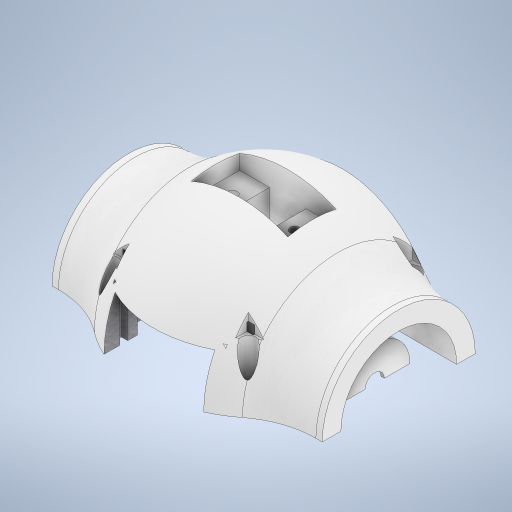
# Autodesk Inventor part: body front moter middle lemon shape for printing
Saved by Autodesk Inventor 2023 (Build 270158000, 158)
## iProperties
Created: 2022-10-08
Part Number: body front moter middle lemon shape for printing
Material: ABS プラスチック
Document SubType Name: Modeling
Designer: ellie
Density: 1.06 g/cm^3
Appearance: 積雪
Author: ellie
Autodesk Inventor part; units mm, degrees
ref_plane "YZ Plane" through (0, 0, 0) normal (1, 0, 0) x (0, 1, 0)
ref_plane "XZ Plane" through (0, 0, 0) normal (0, 1, 0) x (-1, 0, 0)
ref_plane "XY Plane" through (0, 0, 0) normal (0, 0, 1) x (1, 0, 0)
sketch "スケッチ1" plane through (0, 0, 0) normal (0, 1, 0) x (-1, 0, 0)
  circle A0 centre (0, 0) radius 37.5
  line L0 (0, 0) -> (0, -37.5)
  line L1 (0, 0) -> (0, 37.5)
  dimension "d0" = 75
  constraints: 4 end point, 2 point on circle, 2 vertical, 1 centre point, 1 coincident
  measures "d0" diameter of A0
revolve "回転1" add sketch "スケッチ1" angle 180 about axis through (0, 0, 0) along (0, 0, 1) picked at (-2.7815, -24.6866) contours L1 L0 A0
sketch "スケッチ5" plane through (0, 0, 0) normal (0, -1, 0) x (1, 0, 0)
  line L0 (-21, -21) -> (21, -21)
  line L1 (21, -21) -> (21, -9)
  line L2 (21, -9) -> (-21, -9)
  line L3 (-21, -9) -> (-21, -21)
  line L4 (-21, -11) -> (-21, -9)
  line L5 (0, 29.25) -> (-17.5, 29.25)
  line L6 (-17.5, 29.25) -> (-17.5, 26.75)
  line L7 (-17.5, 26.75) -> (0, 26.75)
  line L8 (0, 26.75) -> (0, 29.25)
  line L9 (0, 23.75) -> (-20.5, 23.75)
  line L10 (-20.5, 23.75) -> (-20.5, 22.25)
  line L11 (-20.5, 22.25) -> (0, 22.25)
  line L12 (0, 22.25) -> (0, 23.75)
  line L13 (0, 16.25) -> (-21.5, 16.25)
  line L14 (-21.5, 16.25) -> (-21.5, 13.75)
  line L15 (-21.5, 13.75) -> (0, 13.75)
  line L16 (0, 13.75) -> (0, 16.25)
  line L17 (0, 7.75) -> (-24, 7.75)
  line L18 (-24, 7.75) -> (-24, 5.25)
  line L19 (-24, 5.25) -> (0, 5.25)
  line L20 (0, 5.25) -> (0, 7.75)
  circle A0 centre (0, 0) radius 37.5 projected
  circle A1 centre (0, 0) radius 37.5 projected
  line L21 (0, 37.5) -> (0, -37.5)
  line L22 (37.5, 0) -> (-37.5, 0)
  line L23 (-33.5, 5.25) -> (-24, 5.25)
  line L24 (-24, 5.25) -> (-24, -5.25)
  line L25 (-24, -5.25) -> (-33.5, -5.25)
  line L26 (-33.5, -5.25) -> (-33.5, 5.25)
  line L27 (-24, -8.0262) -> (-24, 5.25)
  line L28 (-29, 23.775) -> (-29, -23.775)
  line L29 (-15.5, 29.25) -> (0, 29.25)
  line L30 (0, 29.25) -> (0, 37.5)
  line L31 (0, 37.5) -> (-15.5, 37.5)
  line L32 (-15.5, 37.5) -> (-15.5, 29.25)
  line L33 (-15.5, 26.75) -> (0, 26.75)
  line L34 (0, 26.75) -> (0, 23.75)
  line L35 (0, 23.75) -> (-15.5, 23.75)
  line L36 (-15.5, 23.75) -> (-15.5, 26.75)
  line L37 (-19, 16.25) -> (0, 16.25)
  line L38 (0, 16.25) -> (0, 22.25)
  line L39 (0, 22.25) -> (-19, 22.25)
  line L40 (-19, 22.25) -> (-19, 16.25)
  line L41 (-19, 13.75) -> (0, 13.75)
  line L42 (0, 13.75) -> (0, 7.75)
  line L43 (0, 7.75) -> (-19, 7.75)
  line L44 (-19, 7.75) -> (-19, 13.75)
  line L45 (-24, 0) -> (-40.9365, 0)
  line L46 (-24, 0) -> (-9.0837, 0)
  line L47 (-9, 5.25) -> (-24, 5.25)
  line L48 (-24, 5.25) -> (-24, -5.25)
  line L49 (-24, -5.25) -> (-9, -5.25)
  line L50 (-9, 5.25) -> (-24, -5.25) construction
  line L51 (-24, 5.25) -> (-9, -5.25) construction
  line L52 (-24, 7.25) -> (-34.5, 7.25)
  line L53 (-34.5, 7.25) -> (-34.5, -7.25)
  line L54 (-34.5, -7.25) -> (-24, -7.25)
  line L55 (-24, -7.25) -> (-24, 7.25)
  line L56 (-24, 7.25) -> (-34.5, -7.25) construction
  line L57 (-34.5, 7.25) -> (-24, -7.25) construction
  line L58 (-8.35, 5.25) -> (-1, 5.25)
  line L59 (-1, 5.25) -> (-1, -5.25)
  line L60 (-1, -5.25) -> (-8.35, -5.25)
  line L61 (-8.35, 5.25) -> (-1, -5.25) construction
  line L62 (-1, 5.25) -> (-8.35, -5.25) construction
  line L63 (-24, 5.25) -> (-29, 5.25)
  line L64 (-24, -5.25) -> (-29, -5.25)
  line L65 (-24, 7.25) -> (-29, 7.25)
  line L66 (-24, -7.25) -> (-29, -7.25)
  line L67 (28.3901, -24.5) -> (-28.3901, -24.5)
  line L68 (-8.35, 5.25) -> (-6.8, 5.25)
  line L69 (-6.6281, -5.25) -> (-7.8281, -5.25)
  line L70 (0, 7.75) -> (1, 7.75)
  line L71 (0, -3) -> (0, 7.75)
  line L72 (-12.5791, -9) -> (-9, -9)
  line L73 (-1, -5.25) -> (-24, -5.25)
  point P0 (0, -21)
  point P1 (0, -9)
  point P2 (0, 28)
  point P3 (0, 23)
  point P4 (0, 15)
  point P5 (0, 6.5)
  point P6 (-21, -15)
  point P7 (-27, -0.5262)
  point P8 (-29, -5.25)
  point P9 (-15.5, 25.25)
  point P10 (-15.5, 34.1467)
  point P11 (0, 29.25)
  point P12 (0, 26.75)
  point P13 (0, 13.75)
  point P14 (0, 16.25)
  point P15 (-29, 0)
  point P16 (-33.5, 0)
  point P17 (-24, 0)
  point P18 (-16.5, 0)
  point P19 (-29.25, 0)
  point P20 (-4.675, 0)
  point P21 (-27, 0.5)
  point P22 (-28, 0.4738)
  point P23 (-28, -11.5262)
  point P24 (-27, -11.5)
  point P25 (-24, -5.25)
  point P26 (-24, -5.25)
  point P27 (-24, -5.25)
  point P28 (-24, 5.25)
  point P29 (-24, -5.25)
  point P30 (-1, 0)
  point P31 (-8, 5.25)
  point P32 (-8, -5.25)
  point P33 (0, 5.25)
  point P34 (-29, -7.25)
  point P35 (-29, 7.25)
  point P36 (-24, -1.3881)
  point P37 (-9, -5.25)
  dimension "d12" = 42
  dimension "d13" = 12
  dimension "d23" = 17.5
  dimension "d24" = 2.5
  dimension "d27" = 20.5
  dimension "d28" = 1.5
  dimension "d30" = 21.5
  dimension "d31" = 2.5
  dimension "d33" = 2.5
  dimension "d88" = 0
  dimension "d89" = 0
  dimension "d90" = 16.5
  dimension "d92" = 21
  dimension "d97" = 9.5
  dimension "d98" = 10.5
  dimension "d113" = 29
  dimension "d122" = 15.5
  dimension "d124" = 3
  dimension "d125" = 15.5
  dimension "d126" = 6
  dimension "d127" = 6
  dimension "d161" = 14.5
  dimension "d162" = 10.5
  dimension "d164" = 10.5
  dimension "d170" = 24.5
  dimension "d187" = 1
  dimension "d283" = 23
  dimension "d284" = 10.5
  dimension "d285" = 15
  dimension "d286" = 34.5
  dimension "d287" = 1
  dimension "d288" = 19
  dimension "d289" = 19
  constraints: 146 end point, 26 parallel, 19 horizontal, 16 midpoint, 16 perpendicular, 15 point on line, 9 collinear, 1 vertical, 20 other
  measures "d12" distance of L2.end L1.end
  measures "d13" distance of L1.end L0.end
  measures "d23" distance of L7.end L6.end
  measures "d24" distance of L6.end L5.end
  measures "d27" distance of L11.end L10.end
  measures "d28" distance of L10.end L9.end
  measures "d30" distance of L15.end L14.end
  measures "d31" distance of L14.end L13.end
  measures "d33" distance of L18.end L17.end
  measures "d89" distance from line of point (0, 0) L22
  measures "d90" distance from line of L0 point (0, -37.5)
  measures "d92" distance of the line from the sketch origin of L3
  measures "d97" distance of L24.end L25.end
  measures "d98" distance of L23.end L24.end
  measures "d113" distance of the line from the sketch origin of L28
  measures "d122" distance of the line from the sketch origin of L32
  measures "d124" distance of L33.end L34.end
  measures "d126" distance of L38.end L37.end
  measures "d127" distance of L41.end L42.end
  measures "d161" distance between parallel lines of L54 L52
  measures "d162" distance between parallel lines of L48 L53
  measures "d164" distance between parallel lines of L60 L58
  measures "d170" distance between parallel lines of L67 L22
  measures "d187" distance between parallel lines of L71 L59
  measures "d283" distance between parallel lines of L55 L59
  measures "d284" distance between parallel lines of L49 L47
  measures "d285" distance of L48.end L49.end
  measures "d286" distance of the line from the sketch origin of L53
  measures "d287" distance of the line from the sketch origin of L59
  measures "d288" distance of the line from the sketch origin of L40
  measures "d289" distance of the line from the sketch origin of L44
extrude "GNSボード" cut sketch "スケッチ5" against normal blind 16.5 contours L8 L7 L6 L5
extrude "GNSボード止めるよう" cut sketch "スケッチ5" against normal blind 15 contours L21 L5 L32 A0 | L21 L9 L36 L7
extrude "アルミ板１" cut sketch "スケッチ5" against normal blind 20.5 contours L12 L11 L10 L9
extrude "メイン基板" cut sketch "スケッチ5" against normal blind 21.5 contours L15 L14 L13 L16
extrude "メイン止めるよう" cut sketch "スケッチ5" against normal blind 16.5 contours L17 L44 L15 L21 | L13 L40 L11 L21
extrude "アルミ板２" cut sketch "スケッチ5" against normal blind 20.5 contours L19 L18 L17 L20
extrude "電池ボックス入れ" cut sketch "スケッチ5" against normal blind 13 contours L3 L2 L21 L0 | L21 L2 L1 L0
extrude "side ut" cut sketch "スケッチ5" against normal blind 100 contours A0 L22 L53 L54 L28 | A0 L28 L52 L53 L22 | L54 L53 L22 L26 L25 L28 | L53 L52 L28 L23 L26 L22 | L25 L26 L22 L28 | L26 L23 L28 L22
extrude "motor case" add sketch "スケッチ5" against normal blind 7 contours L54 L53 L22 L26 L25 L28 | L28 L25 L27 L54 | L53 L52 L28 L23 L26 L22 | L28 L22 L24 L25 | L25 L26 L22 L28 | L22 L28 L23 L24 | L52 L18 L23 L28 | L26 L23 L28 L22
extrude "bottom cut" cut sketch "スケッチ5" against normal blind 90 contours L67 A0 L21 | L21 A0 L67
extrude "motor" cut sketch "スケッチ5" against normal blind 6 contours L28 L22 L24 L25 | L25 L26 L22 L28 | L22 L28 L23 L24 | L26 L23 L28 L22
extrude "motor block" cut sketch "スケッチ5" against normal up to surface (6 mm away) contours L59 L60 L73 L49 L24 L22 | L22 L24 L19 L59
sketch "スケッチ26" plane through (-34.5, 0, -7.25) normal (-1, 0, 0) x (0, 0, 1)
  line L0 (14.5, 0) -> (0, 0) projected
  circle A0 centre (7.25, 0) radius 3
  point P0 (7.25, 0)
  point P1 (7.25, 0)
  point P2 (4.25, 0)
  point P3 (10.25, 0)
  dimension "d197" = 6
  constraints: 1 centre point, 1 coincident
  measures "d197" diameter of A0
extrude "押し出し34" cut sketch "スケッチ26" against normal blind 27 contours L0 A0 picked at (7.9985, 0.6631)
mirror "ミラー11" about plane through (0, 0, 0) normal (1, 0, 0) of "GNSボード", "GNSボード止めるよう", "アルミ板１", "メイン止めるよう", "メイン基板", "アルミ板２", "motor", "押し出し34", "motor case", "電池ボックス入れ", "motor block", "side ut"
ref_plane "作業平面5" through (0, 13, 0) normal (0, -1, 0) x (1, 0, 0)
ref_plane "作業平面6" through (-15.5, 37, 29.25) normal (0, -1, 0) x (1, 0, 0)
sketch "スケッチ29" plane through (-15.5, 37, 29.25) normal (0, -1, 0) x (1, 0, 0)
  line L0 (15.5, -29.25) -> (-67.7134, -29.25)
  line L1 (-67.7134, -29.25) -> (15.5, -29.25)
  line L2 (110.7852, -24.5555) -> (110.7852, -27.3413)
  line L3 (15.5, -29.25) -> (98.1975, -29.25)
  circle A0 centre (25.2, -29.25) radius 1.5
  circle A1 centre (5.8, -29.25) radius 1.5
  line L4 (32.1864, 0) -> (-1.1864, 0) projected
  line L5 (15.5, 0) -> (15.5, -53.75)
  line L6 (-12.8901, -53.75) -> (43.8901, -53.75) projected
  point P0 (32.5, 0)
  point P1 (-1.5, 0)
  point P2 (43.8901, -53.75)
  point P3 (-11.5, -52)
  point P4 (42.5, -52)
  dimension "d205" = 3
  dimension "d206" = 19.4
  dimension "d207" = 0
  constraints: 10 end point, 2 centre point, 2 horizontal, 1 collinear, 1 midpoint, 1 vertical, 3 other
  measures "d205" diameter of A0
  measures "d206" distance of A1.centre A0.centre
  measures "d207" distance from line of L3 A0.centre
extrude "押し出し36" cut sketch "スケッチ29" along normal blind 25
sketch "スケッチ30" plane through (-15.5, 37, 29.25) normal (0, -1, 0) x (1, 0, 0)
  line L0 (0.5, -21.75) -> (30.5, -21.75)
  line L1 (30.5, -21.75) -> (30.5, -36.75)
  line L2 (30.5, -36.75) -> (0.5, -36.75)
  line L3 (0.5, -36.75) -> (0.5, -21.75)
  line L4 (0.5, -21.75) -> (30.5, -36.75) construction
  line L5 (30.5, -21.75) -> (0.5, -36.75) construction
  point P0 (15.5, -29.25)
  dimension "d210" = 30
  dimension "d211" = 15
  constraints: 12 end point, 2 midpoint, 2 parallel, 1 horizontal, 1 perpendicular
  measures "d210" distance of L1.end L2.end
  measures "d211" distance of L0.end L1.end
extrude "押し出し37" cut sketch "スケッチ30" along normal mid plane 16
ref_plane "作業平面7" through (-15.5, 12, 29.25) normal (0, 1, 0) x (1, 0, 0)
sketch "スケッチ33" plane through (-15.5, 12, 29.25) normal (0, 1, 0) x (1, 0, 0)
  circle A0 centre (25.2, 29.25) radius 1.5 projected
  circle A1 centre (5.8, 29.25) radius 1.5 projected
  line L0 (0.5, 36.75) -> (0.5, 21.75) projected
  line L1 (30.5, 21.75) -> (30.5, 36.75) projected
  line L2 (0.5, 21.75) -> (30.5, 21.75) projected
  line L3 (30.5, 36.75) -> (0.5, 36.75) projected
  line L4 (15.5, 0) -> (15.5, 53.75) projected
  line L5 (15.5, 29.25) -> (98.1975, 29.25) projected
  circle A2 centre (25.2, 29.25) radius 3
  circle A3 centre (5.8, 29.25) radius 3
  dimension "d219" = 6
  dimension "d220" = 6
  constraints: 2 centre point, 2 coincident
  measures "d219" diameter of A2
  measures "d220" diameter of A3
extrude "押し出し39" cut sketch "スケッチ33" along normal blind 10 contours L5 A0 | L5 A2 A0 | A0 L5 A2 | A0 L5 | A1 | A3
sketch "スケッチ35" plane through (-17.5, 0, 26.75) normal (0, -1, 0) x (1, 0, 0)
  circle A0 centre (-4, -0.5) radius 2.4
  line L0 (-16, -21.5) -> (-6.5, -21.5) projected
  line L1 (-16, -32) -> (-16, -21.5) projected
  line L2 (16.5, -32) -> (-16, -32) projected
  line L3 (-17, -23.75) -> (-16, -23.75) projected
  line L4 (-16, -23.75) -> (-16, -21.5) projected
  line L5 (-16, -21.5) -> (-6.5, -21.5) projected
  line L6 (-6.5, -21.5) -> (-6.5, -19) projected
  line L7 (-6.5, -19) -> (-1.5, -19) projected
  line L8 (-1.5, -19) -> (-1.5, -13) projected
  line L9 (-1.5, -13) -> (-4, -13) projected
  line L10 (-4, -13) -> (-4, -10.5) projected
  line L11 (-4, -10.5) -> (-1.5, -10.5) projected
  line L12 (-1.5, -10.5) -> (-1.5, -4.5) projected
  line L13 (-1.5, -4.5) -> (-3, -4.5) projected
  line L14 (-3, -4.5) -> (-3, -3) projected
  line L15 (-3, -3) -> (2, -3) projected
  line L16 (2, -3) -> (2, 0) projected
  line L17 (2, 0) -> (0, 0) projected
  line L18 (0, 0) -> (0, 2.5) projected
  line L19 (0, 2.5) -> (2, 2.5) projected
  line L20 (2, 2.5) -> (2, 7.3967) projected
  arc A1 (2, 7.3967) -> (-11.5, -2.975) centre (17.5, -26.75) ccw projected
  line L21 (-11.5, -2.975) -> (-11.5, -19.5) projected
  line L22 (-11.5, -19.5) -> (-17, -19.5) projected
  line L23 (-17, -19.5) -> (-17, -23.75) projected
  line L24 (16.5, -32) -> (16.5, -21.5) projected
  line L25 (-6.5, -21.5) -> (16.5, -21.5) projected
  point P0 (-16, -23.75)
  dimension "d231" = 4.8
  dimension "d234" = 4
  dimension "d300" = 2.5
  constraints: 1 centre point
  measures "d231" diameter of A0
  measures "d234" distance from line of A0.centre L18
  measures "d300" distance from line of A0.centre L15
extrude "押し出し41" cut sketch "スケッチ35" against normal blind 20 contours A0
mirror "ミラー12" about plane through (0, 0, 0) normal (1, 0, 0) of "押し出し41"
sketch "スケッチ36" plane through (-34.5, 0, -7.25) normal (0, -1, 0) x (1, 0, 0)
  circle A0 centre (9.5, -14) radius 2.4
  line L0 (35.5, 12.5) -> (33.5, 12.5) projected
  line L1 (10.5, 12.5) -> (10.5, 15) projected
  line L2 (1, 2) -> (1, 4.25) projected
  line L3 (1, 4.25) -> (0, 4.25) projected
  line L4 (0, 4.25) -> (0, 0) projected
  line L5 (0, 0) -> (5.5, 0) projected
  line L6 (5.5, 0) -> (5.5, -16.525) projected
  arc A1 (5.5, -16.525) -> (6.1099, -17.25) centre (34.5, 7.25) ccw projected
  line L7 (6.1099, -17.25) -> (62.8901, -17.25) projected
  arc A2 (62.8901, -17.25) -> (63.5, -16.525) centre (34.5, 7.25) ccw projected
  line L8 (63.5, -16.525) -> (63.5, 0) projected
  line L9 (69, 0) -> (63.5, 0) projected
  line L10 (69, 4.25) -> (69, 0) projected
  line L11 (69, 4.25) -> (68, 4.25) projected
  line L12 (68, 4.25) -> (68, 2) projected
  line L13 (58.5, 15) -> (58.5, 12.5) projected
  line L14 (13.5, -1.75) -> (55.5, -1.75) projected
  line L15 (55.5, -1.75) -> (55.5, -13.75) projected
  line L16 (55.5, -13.75) -> (13.5, -13.75) projected
  line L17 (13.5, -13.75) -> (13.5, -1.75) projected
  line L18 (55.5, -1.75) -> (55.5, -13.75) projected
  line L19 (13.5, -1.75) -> (55.5, -1.75) projected
  line L20 (13.5, -13.75) -> (13.5, -1.75) projected
  line L21 (55.5, -13.75) -> (13.5, -13.75) projected
  line L22 (0, 10.25) -> (1, 10.25) projected
  line L23 (1, 10.25) -> (1, 12.5) projected
  line L24 (1, 12.5) -> (10.5, 12.5) projected
  line L25 (10.5, 15) -> (15.5, 15) projected
  line L26 (15.5, 15) -> (15.5, 21) projected
  line L27 (15.5, 21) -> (13, 21) projected
  line L28 (13, 21) -> (13, 23.5) projected
  line L29 (13, 23.5) -> (15.5, 23.5) projected
  line L30 (15.5, 23.5) -> (15.5, 29.5) projected
  line L31 (15.5, 29.5) -> (14, 29.5) projected
  line L32 (14, 29.5) -> (14, 31) projected
  line L33 (14, 31) -> (19, 31) projected
  line L34 (19, 31) -> (19, 34) projected
  line L35 (19, 34) -> (17, 34) projected
  line L36 (17, 34) -> (17, 36.5) projected
  line L37 (17, 36.5) -> (19, 36.5) projected
  line L38 (19, 36.5) -> (19, 41.3967) projected
  line L39 (5.5, 31.025) -> (5.5, 14.5) projected
  line L40 (5.5, 14.5) -> (0, 14.5) projected
  line L41 (0, 14.5) -> (0, 10.25) projected
  line L42 (33.5, 2) -> (1, 2) projected
  line L43 (68, 2) -> (35.5, 2) projected
  line L44 (68, 10.25) -> (69, 10.25) projected
  line L45 (69, 14.5) -> (69, 10.25) projected
  line L46 (63.5, 14.5) -> (69, 14.5) projected
  line L47 (63.5, 14.5) -> (63.5, 31.025) projected
  line L48 (50, 41.3967) -> (50, 36.5) projected
  line L49 (50, 36.5) -> (52, 36.5) projected
  line L50 (52, 36.5) -> (52, 34) projected
  line L51 (52, 34) -> (50, 34) projected
  line L52 (50, 34) -> (50, 31) projected
  line L53 (50, 31) -> (55, 31) projected
  line L54 (55, 31) -> (55, 29.5) projected
  line L55 (55, 29.5) -> (53.5, 29.5) projected
  line L56 (53.5, 29.5) -> (53.5, 23.5) projected
  line L57 (53.5, 23.5) -> (56, 23.5) projected
  line L58 (56, 23.5) -> (56, 21) projected
  line L59 (56, 21) -> (53.5, 21) projected
  line L60 (53.5, 21) -> (53.5, 15) projected
  line L61 (53.5, 15) -> (58.5, 15) projected
  line L62 (58.5, 12.5) -> (68, 12.5) projected
  line L63 (68, 12.5) -> (68, 10.25) projected
  circle A3 centre (13, 33.5) radius 2.4 projected
  circle A4 centre (56, 33.5) radius 2.4 projected
  arc A5 (19, 41.3967) -> (5.5, 31.025) centre (34.5, 7.25) ccw projected
  arc A6 (63.5, 31.025) -> (50, 41.3967) centre (34.5, 7.25) ccw projected
  line L64 (35.5, 2) -> (35.5, 12.5) projected
  line L65 (33.5, 12.5) -> (33.5, 2) projected
  dimension "d237" = 4.8
  dimension "d238" = 4
  dimension "d299" = 16
  constraints: 1 centre point
  measures "d237" diameter of A0
  measures "d238" distance from line of A0.centre L17
  measures "d299" distance from line of A0.centre L42
extrude "押し出し42" cut sketch "スケッチ36" against normal blind 25 contours A0
mirror "ミラー13" about plane through (0, 0, 0) normal (1, 0, 0) of "押し出し42"
ref_plane "作業平面8" through (-17.5, 35, 26.75) normal (0, -1, 0) x (1, 0, 0)
sketch "スケッチ37" plane through (-17.5, 35, 26.75) normal (0, -1, 0) x (1, 0, 0)
  line L0 (39, -10.5) -> (-4, -10.5) projected
  line L1 (2.5, -19.25) -> (2.5, -34.25) projected
  line L2 (32.5, -34.25) -> (32.5, -19.25) projected
  arc A0 (33, 3.9257) -> (2, 3.9257) centre (17.5, -26.75) ccw projected
  line L3 (33, 3.9257) -> (33, 7.3967) projected
  line L4 (46.5, -2.975) -> (46.5, -50.525) projected
  arc A1 (45.8901, -51.25) -> (46.5, -50.525) centre (17.5, -26.75) ccw projected
  line L5 (45.8901, -51.25) -> (-10.8901, -51.25) projected
  arc A2 (-11.5, -50.525) -> (-10.8901, -51.25) centre (17.5, -26.75) ccw projected
  line L6 (-11.5, -50.525) -> (-11.5, -2.975) projected
  line L7 (2, 7.3967) -> (2, 3.9257) projected
  line L8 (-7, 2.5) -> (-1, 2.5)
  line L9 (-1, 2.5) -> (-1, -3.5)
  line L10 (-1, -3.5) -> (-7, -3.5)
  line L11 (-7, -3.5) -> (-7, 2.5)
  arc A3 (37.6, -40) -> (37.6, -40) centre (-4, -0.5) ccw projected
  line L12 (-7, 2.5) -> (-1, -3.5) construction
  line L13 (-1, 2.5) -> (-7, -3.5) construction
  line L14 (42, 2.5) -> (36, 2.5)
  line L15 (36, 2.5) -> (36, -3.5)
  line L16 (36, -3.5) -> (42, -3.5)
  line L17 (42, -3.5) -> (42, 2.5)
  arc A4 (37.6, -40) -> (37.6, -40) centre (39, -0.5) ccw projected
  line L18 (42, 2.5) -> (36, -3.5) construction
  line L19 (36, 2.5) -> (42, -3.5) construction
  line L20 (-4.5, -45) -> (-10.5, -45)
  line L21 (-10.5, -45) -> (-10.5, -51)
  line L22 (-10.5, -51) -> (-4.5, -51)
  line L23 (-4.5, -51) -> (-4.5, -45)
  circle A5 centre (-7.5, -48) radius 2.4 projected
  line L24 (-4.5, -45) -> (-10.5, -51) construction
  line L25 (-10.5, -45) -> (-4.5, -51) construction
  line L26 (45.5, -45) -> (39.5, -45)
  line L27 (39.5, -45) -> (39.5, -51)
  line L28 (39.5, -51) -> (45.5, -51)
  line L29 (45.5, -51) -> (45.5, -45)
  circle A6 centre (42.5, -48) radius 2.4 projected
  line L30 (45.5, -45) -> (39.5, -51) construction
  line L31 (39.5, -45) -> (45.5, -51) construction
  line L32 (32.5, -19.25) -> (2.5, -19.25) projected
  line L33 (2.5, -34.25) -> (32.5, -34.25) projected
  arc A7 (46.5, -2.975) -> (33, 7.3967) centre (17.5, -26.75) ccw projected
  arc A8 (2, 7.3967) -> (-11.5, -2.975) centre (17.5, -26.75) ccw projected
  point P0 (-1.6, 0.4)
  point P1 (35.6, 0.4)
  point P2 (-3.6, -40)
  point P3 (36.5, 1.5)
  point P4 (-2.5, 1.5)
  dimension "d243" = 6
  dimension "d244" = 6
  dimension "d245" = 6
  dimension "d246" = 6
  dimension "d247" = 6
  dimension "d248" = 6
  dimension "d249" = 6
  dimension "d250" = 6
  constraints: 48 end point, 8 midpoint, 8 parallel, 4 horizontal, 4 perpendicular, 10 other
  measures "d243" distance of L9.end L10.end
  measures "d244" distance of L8.end L9.end
  measures "d245" distance of L16.end L15.end
  measures "d246" distance of L15.end L14.end
  measures "d247" distance of L22.end L21.end
  measures "d248" distance of L21.end L20.end
  measures "d249" distance of L28.end L27.end
  measures "d250" distance of L27.end L26.end
extrude "押し出し43" cut sketch "スケッチ37" along normal blind 20 contours L23 L22 L21 L20 | A5 | L29 L28 L27 L26 | A6
extrude "押し出し44" cut sketch "スケッチ37" along normal blind 17 contours A8 L11 L8 | L8 L9 L10 L11 A8 | A7 L14 L17 | L17 L16 L15 L14 A7
sketch "スケッチ39" plane through (-15.5, 29, 29.25) normal (0, 1, 0) x (1, 0, 0)
  line L0 (21.2, 21.75) -> (9.8, 21.75)
  line L1 (9.8, 21.75) -> (9.8, 36.75)
  line L2 (9.8, 36.75) -> (21.2, 36.75)
  line L3 (21.2, 36.75) -> (21.2, 21.75)
  line L4 (21.2, 21.75) -> (9.8, 36.75) construction
  line L5 (9.8, 21.75) -> (21.2, 36.75) construction
  circle A0 centre (5.8, 29.25) radius 1.5 projected
  circle A1 centre (25.2, 29.25) radius 1.5 projected
  line L6 (0.5, 21.75) -> (30.5, 21.75) projected
  line L7 (30.5, 36.75) -> (0.5, 36.75) projected
  circle A2 centre (5.8, 29.25) radius 1.5 projected
  circle A3 centre (25.2, 29.25) radius 1.5 projected
  line L8 (0.5, 36.75) -> (30.5, 36.75) projected
  line L9 (0.5, 21.75) -> (0.5, 36.75) projected
  line L10 (30.5, 21.75) -> (0.5, 21.75) projected
  line L11 (30.5, 36.75) -> (30.5, 21.75) projected
  point P0 (15.5, 29.25)
  dimension "d255" = 4
  dimension "d256" = 0
  constraints: 12 end point, 2 midpoint, 2 parallel, 1 horizontal, 1 perpendicular
  measures "d255" distance from line of L1 A0.centre
  measures "d256" distance between parallel lines of L6 L0
extrude "押し出し45" cut sketch "スケッチ39" against normal up to surface (12.5 mm away) contours L0 L1 L2 L3
ref_plane "作業平面9" through (42, 0, -7.25) normal (1, 0, 0) x (0, 0, -1)
sketch "スケッチ41" plane through (42, 0, -7.25) normal (1, 0, 0) x (0, 0, -1)
  arc A0 (-4.25, 0) -> (-10.25, 0) centre (-7.25, 0) ccw projected
  arc A1 (-4.25, 0) -> (-10.25, 0) centre (-7.25, 0) ccw projected
  line L0 (-4.25, 0) -> (0, 0) projected
  line L1 (0, 0) -> (0, 7) projected
  line L2 (0, 7) -> (-14.5, 7) projected
  line L3 (-14.5, 0) -> (-14.5, 7) projected
  line L4 (-14.5, 0) -> (-10.25, 0) projected
  line L5 (0, 7) -> (0, 0) projected
  line L6 (16.525, 0) -> (0, 0) projected
  arc A2 (16.525, 0) -> (-31.025, 0) centre (-7.25, 0) ccw projected
  line L7 (-14.5, 0) -> (-31.025, 0) projected
  line L8 (-14.5, 0) -> (-14.5, 7) projected
  line L9 (-14.5, 7) -> (0, 7) projected
  line L10 (-2, 0) -> (-12, 0) projected
  line L11 (-2, 0) -> (-2, 6) projected
  line L12 (-12, 6) -> (-2, 6) projected
  line L13 (-12, 0) -> (-12, 6) projected
  circle A3 centre (-7.25, 0) radius 23
  circle A4 centre (-7.25, 0) radius 18
  point P0 (-25.25, 0)
  point P1 (10.75, 0)
  dimension "d267" = 46
  dimension "d268" = 36
  constraints: 2 centre point, 2 coincident
  measures "d267" diameter of A3
  measures "d268" diameter of A4
extrude "押し出し47" add sketch "スケッチ41" against normal up to surface (13 mm away) contours A4 L7 A3 L6 | A3 L7 A2 L6 picked at (-28.1862, 3.2706)
fillet "面フィレット1" radius 27.7 1 edges at (29, 23.775, 0)
mirror "ミラー14" about plane through (0, 0, 0) normal (1, 0, 0) of "面フィレット1", "押し出し47"
sketch "スケッチ42" plane through (0, 16.5, 0) normal (0, -1, 0) x (1, 0, 0)
  line L0 (-5.7, 7.5) -> (5.7, 7.5) projected
  line L1 (-5.7, 5.25) -> (-5.7, 7.5) projected
  line L2 (5.7, 7.5) -> (5.7, 5.25) projected
  line L3 (15, 7.5) -> (5.7, 7.5) projected
  line L4 (5.7, 7.5) -> (-5.7, 7.5)
  line L5 (-5.7, 7.5) -> (-5.7, 10.5)
  line L6 (-5.7, 10.5) -> (5.7, 10.5)
  line L7 (5.7, 10.5) -> (5.7, 7.5)
  point P0 (0, 0)
  point P1 (-5.7, 7.25)
  point P2 (5.7, 7.25)
  point P3 (-5.7, 7.5)
  dimension "d272" = 3
  constraints: 8 end point, 3 parallel, 1 horizontal, 1 perpendicular
  measures "d272" distance of L6.end L0.end
extrude "押し出し48" cut sketch "スケッチ42" against normal blind 10
sketch "スケッチ43" plane through (34.5, 0, -3) normal (1, 0, 0) x (0, 0, -1)
  arc A0 (0, 0) -> (-6, 0) centre (-3, 0) ccw projected
  circle A1 centre (-3, 0) radius 11
  arc A2 (15, 0) -> (-21, 0) centre (-3, 0) ccw projected
  line L0 (-10.25, 0) -> (-21, 0) projected
  line L1 (-10.25, 0) -> (-10.25, 7) projected
  line L2 (-10.25, 7) -> (4.25, 7) projected
  line L3 (4.25, 7) -> (4.25, 0) projected
  line L4 (15, 0) -> (4.25, 0) projected
  line L5 (-10.25, 0) -> (-6, 0) projected
  line L6 (0, 0) -> (4.25, 0) projected
  line L7 (2, 0) -> (-8, 0) projected
  point P0 (-3, 0)
  point P1 (8, 0)
  point P2 (-14, 0)
  dimension "d275" = 22
  constraints: 1 centre point, 1 coincident
  measures "d275" diameter of A1
extrude "押し出し49" add sketch "スケッチ43" against normal up to surface (5.5 mm away) contours L3 L2 L1 L0 A1 L4
mirror "ミラー15" about plane through (0, 0, 0) normal (1, 0, 0) of "押し出し49"
sketch "スケッチ44" plane through (-34.5, 0, 0) normal (-1, 0, 0) x (0, 0, 1)
  point P0 (0, 0)
sketch "スケッチ45" plane through (-29, 0, 0) normal (-1, 0, 0) x (0, 0, 1)
  circle A0 centre (0, 0) radius 11
  arc A1 (3, 0) -> (-3, 0) centre (0, 0) ccw projected
  circle A2 centre (0, 0) radius 18
  line L0 (18, 0) -> (11, 0) projected
  line L1 (-11, 0) -> (-18, 0) projected
  point P0 (0, 0)
  dimension "d278" = 22
  dimension "d279" = 36
  constraints: 2 centre point, 2 coincident
  measures "d278" diameter of A0
  measures "d279" diameter of A2
extrude "押し出し50" cut sketch "スケッチ45" against normal blind 5 contours A0 L1 A2 L0 picked at (-15.4923, 1.4359)
mirror "ミラー16" about plane through (0, 0, 0) normal (1, 0, 0) of "押し出し50"
sketch "スケッチ46" plane through (-33.5, 0, -5.25) normal (0, -1, 0) x (1, 0, 0)
  line L0 (32.5, 0) -> (32.5, 10.5) projected
  line L1 (67, 0) -> (34.5, 0) projected
  line L2 (32.5, 10.5) -> (34.5, 10.5)
  line L3 (34.5, 10.5) -> (34.5, 0)
  line L4 (34.5, 0) -> (32.5, 0)
  line L5 (32.5, 0) -> (32.5, 10.5)
  point P0 (33.5, 5.25)
  constraints: 8 end point, 2 parallel, 1 horizontal, 1 perpendicular
extrude "押し出し51" cut sketch "スケッチ46" against normal up to surface (6 mm away)
sketch "スケッチ47" plane through (0, 6, 0) normal (0, -1, 0) x (1, 0, 0)
  line L0 (-27, 5.25) -> (-25.5, 5.25)
  line L1 (-25.5, 5.25) -> (-25.5, 2.25)
  line L2 (-25.5, 2.25) -> (-27, 2.25)
  line L3 (-27, 2.25) -> (-27, 5.25)
  line L4 (-33.5, 3) -> (-33.5, 5.25) projected
  line L5 (-33.5, 5.25) -> (-24, 5.25) projected
  point P0 (0, 0)
  dimension "d293" = 6.5
  dimension "d294" = 8
  dimension "d295" = 3
  constraints: 8 end point, 2 parallel, 1 collinear, 1 horizontal, 1 perpendicular
  measures "d293" distance between parallel lines of L4 L3
  measures "d294" distance between parallel lines of L4 L1
  measures "d295" distance of L0.end L1.end
extrude "押し出し52" add sketch "スケッチ47" along normal blind 6
